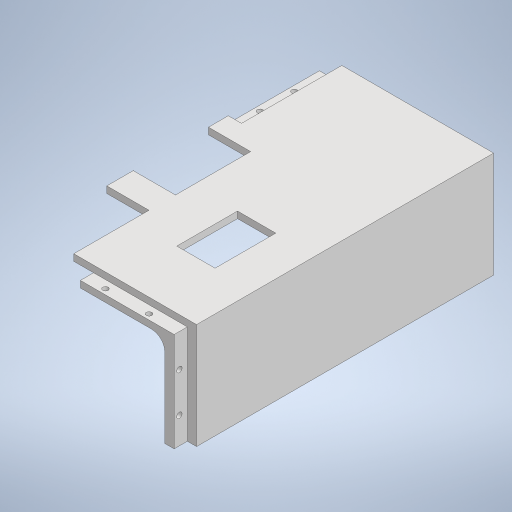
# Autodesk Inventor part: top_4
Saved by Autodesk Inventor 2023 (Build 270158000, 158)
## iProperties
Created: 2024-04-26
Part Number: top_4
Material: 常规
Document SubType Name: Modeling
Designer: Nitrene.P.L
Density: 1 g/cm^3
Appearance: 默认
Author: Nitrene.P.L
Autodesk Inventor part; units mm, degrees
ref_plane "YZ Plane" through (0, 0, 0) normal (1, 0, 0) x (0, 1, 0)
ref_plane "XZ Plane" through (0, 0, 0) normal (0, 1, 0) x (-1, 0, 0)
ref_plane "XY Plane" through (0, 0, 0) normal (0, 0, 1) x (1, 0, 0)
sketch "草图7" plane through (0, 0, 0) normal (0, 1, 0) x (-1, 0, 0)
  line L0 (125, 235) -> (-125, 235)
  line L1 (-125, 235) -> (-125, -235)
  line L2 (-125, -235) -> (125, -235)
  line L3 (125, -235) -> (125, 235)
  line L4 (0, 3) -> (0, -5)
  line L5 (3.5058, 0) -> (-3.4421, 0)
  line L6 (25, 144) -> (-32, 144)
  line L7 (-32, 144) -> (-32, 87)
  line L8 (-32, 87) -> (25, 87)
  line L9 (25, 87) -> (25, 144)
  line L10 (25, 67) -> (-32, 67)
  line L11 (-32, 67) -> (-32, 10)
  line L12 (-32, 10) -> (25, 10)
  line L13 (25, 10) -> (25, 67)
  line L14 (25, -10) -> (-32, -10)
  line L15 (-32, -10) -> (-32, -67)
  line L16 (-32, -67) -> (25, -67)
  line L17 (25, -67) -> (25, -10)
  line L18 (25, -87) -> (-32, -87)
  line L19 (-32, -87) -> (-32, -144)
  line L20 (-32, -144) -> (25, -144)
  line L21 (25, -144) -> (25, -87)
  line L22 (-66, 100) -> (-95, 100)
  line L23 (-95, 100) -> (-95, 54)
  line L24 (-95, 54) -> (-66, 54)
  line L25 (-66, 54) -> (-66, 100)
  line L26 (-66, -54) -> (-95, -54)
  line L27 (-95, -54) -> (-95, -100)
  line L28 (-95, -100) -> (-66, -100)
  line L29 (-66, -100) -> (-66, -54)
  line L30 (100, 15) -> (70, 15)
  line L31 (70, 15) -> (70, -15)
  line L32 (70, -15) -> (100, -15)
  line L33 (100, -15) -> (100, 15)
  circle A0 centre (65, 182) radius 10
  circle A1 centre (65, -182) radius 10
  circle A2 centre (65, 182) radius 15
  circle A3 centre (80, 182) radius 1.5
  circle A4 centre (57.5, 194.9904) radius 1.5
  circle A5 centre (57.5, 169.0096) radius 1.5
  line L34 (125, 235) -> (0, 235)
  line L35 (0, 235) -> (0, 0)
  line L36 (0, 0) -> (125, 0)
  line L37 (125, 0) -> (125, 235)
  line L38 (-125, 235) -> (0, 235)
  line L39 (0, 235) -> (0, 0)
  line L40 (0, 0) -> (-125, 0)
  line L41 (-125, 0) -> (-125, 235)
  line L42 (-125, -235) -> (0, -235)
  line L43 (0, -235) -> (0, 0)
  line L44 (0, 0) -> (-125, 0)
  line L45 (-125, 0) -> (-125, -235)
  line L46 (125, -235) -> (0, -235)
  line L47 (0, -235) -> (0, 0)
  line L48 (0, 0) -> (125, 0)
  line L49 (125, 0) -> (125, -235)
  circle A6 centre (65, -182) radius 15
  circle A7 centre (80, -182) radius 1.5
  circle A8 centre (57.5, -169.0096) radius 1.5
  circle A9 centre (57.5, -194.9904) radius 1.5
  point P0 (0, -87)
  point P1 (0, -67)
  point P2 (0, -10)
  point P3 (0, -235)
  point P4 (0, -144)
  dimension "d115" = 30
  dimension "d118" = 30
  dimension "d84" = 470
  dimension "d85" = 250
  dimension "d86" = 57
  dimension "d87" = 57
  dimension "d88" = 57
  dimension "d89" = 57
  dimension "d90" = 57
  dimension "d91" = 57
  dimension "d92" = 57
  dimension "d93" = 57
  dimension "d94" = 91
  dimension "d95" = 20
  dimension "d96" = 20
  dimension "d97" = 20
  dimension "d98" = 93
  dimension "d99" = 29
  dimension "d100" = 46
  dimension "d101" = 46
  dimension "d102" = 135
  dimension "d103" = 108
  dimension "d104" = 30
  dimension "d105" = 30
  dimension "d106" = 30
  dimension "d107" = 25
  dimension "d108" = 220
  dimension "d109" = 20
  dimension "d110" = 53
  dimension "d111" = 60
  dimension "d112" = 20
  dimension "d113" = 53
  dimension "d114" = 60
  dimension "d116" = 3
  dimension "d117" = 360
  dimension "d119" = 3
  dimension "d120" = 360
  constraints: 100 end point, 24 parallel, 14 horizontal, 12 perpendicular, 8 centre point, 3 collinear, 2 coincident, 2 horizontal alignment, 2 point on line, 2 vertical, 20 other
  measures "d84" distance of L3.start L37.end
  measures "d85" distance of L37.end L1.start
  measures "d86" distance of L8.end L8.start
  measures "d87" distance of L8.start L6.end
  measures "d88" distance of L12.end L12.start
  measures "d89" distance of L12.start L10.end
  measures "d90" distance of L16.end L16.start
  measures "d91" distance of L16.start L14.end
  measures "d92" distance of L20.end L20.start
  measures "d93" distance of L20.start L19.start
  measures "d94" distance between parallel lines of L0 L6
  measures "d95" distance between parallel lines of L10 L8
  measures "d96" distance between parallel lines of L12 L14
  measures "d97" distance between parallel lines of L18 L16
  measures "d98" distance between parallel lines of L1 L7
  measures "d99" distance of L25.start L23.end
  measures "d100" distance of L23.end L22.end
  measures "d101" distance of L28.start L27.start
  measures "d102" distance between parallel lines of L0 L22
  measures "d103" distance between parallel lines of L26 L24
  measures "d104" distance between parallel lines of L1 L23
  measures "d105" distance of L33.start L31.end
  measures "d106" distance of L31.end L30.end
  measures "d107" distance between parallel lines of L3 L33
  measures "d108" distance between parallel lines of L0 L30
  measures "d109" diameter of A0
  measures "d110" distance from line of L0 A0.centre
  measures "d111" distance from line of L3 A0.centre
  measures "d112" diameter of A1
  measures "d113" distance from line of L2 A1.centre
  measures "d114" distance from line of L3 A1.centre
  measures "d116" diameter of A3
  measures "d119" diameter of A7
extrude "拉伸7" add sketch "草图7" along normal blind 10 contours L40 L5 L4 L43 L14 L15 L16 L18 L19 L20 L2 L1
sketch "草图8" plane through (0, 0, 0) normal (0, -1, 0) x (1, 0, 0)
  line L0 (0, 0) -> (125, 0) projected
  line L1 (0, -235) -> (0, -144) projected
  line L2 (47, 0) -> (0, 0)
  line L3 (0, 0) -> (0, -159)
  line L4 (0, -159) -> (47, -159)
  line L5 (47, -159) -> (47, 0)
  line L6 (32, -67) -> (32, -10) projected
  line L7 (0, -144) -> (32, -144) projected
  line L8 (111, -39) -> (47, -39)
  line L9 (47, -39) -> (47, -115)
  line L10 (47, -115) -> (111, -115)
  line L11 (111, -115) -> (111, -39)
  line L12 (95, -54) -> (66, -54) projected
  line L13 (66, -100) -> (95, -100) projected
  line L14 (95, -100) -> (95, -54) projected
  line L15 (66, -54) -> (66, -100) projected
  dimension "d123" = 15
  dimension "d124" = 15
  dimension "d125" = 15
  dimension "d126" = 15
  dimension "d127" = 16
  dimension "d128" = 19
  constraints: 16 end point, 4 parallel, 2 horizontal, 2 perpendicular, 2 point on line
  measures "d123" distance between parallel lines of L6 L5
  measures "d124" distance between parallel lines of L7 L4
  measures "d125" distance between parallel lines of L8 L12
  measures "d126" distance between parallel lines of L13 L10
  measures "d127" distance between parallel lines of L14 L11
  measures "d128" distance between parallel lines of L9 L15
extrude "拉伸8" cut sketch "草图8" against normal blind 5
sketch "草图9" plane through (0, 0, 0) normal (0, -1, 0) x (1, 0, 0)
  line L0 (125, -235) -> (0, -235) projected
  line L1 (125, 0) -> (111, 0)
  line L2 (111, 0) -> (111, -235)
  line L3 (111, -235) -> (125, -235)
  line L4 (125, -235) -> (125, 0)
  line L5 (0, -235) -> (0, -159) projected
  line L6 (125, 0) -> (125, -235) projected
  line L7 (0, -235) -> (125, -235)
  line L8 (125, -235) -> (125, -221)
  line L9 (125, -221) -> (0, -221)
  line L10 (0, -221) -> (0, -235)
  point P0 (0, 0)
  point P1 (111, -221)
  dimension "d131" = 14
  dimension "d132" = 14
  constraints: 16 end point, 4 parallel, 2 horizontal, 2 perpendicular, 2 point on line
  measures "d131" distance of L3.end L2.end
  measures "d132" distance of L8.end L7.end
extrude "拉伸9" add sketch "草图9" along normal blind 70
sketch "草图10" plane through (0, 10, 0) normal (0, 1, 0) x (1, 0, 0)
  line L0 (0, 221) -> (0, 159) projected
  line L1 (125, 235) -> (0, 235) projected
  line L2 (0, 159) -> (10, 159)
  line L3 (10, 159) -> (10, 235)
  line L4 (10, 235) -> (0, 235)
  line L5 (0, 235) -> (0, 159)
  point P0 (0, 0)
  dimension "d135" = 10
  constraints: 8 end point, 2 parallel, 1 horizontal, 1 perpendicular, 1 point on line
  measures "d135" distance of L4.end L3.end
extrude "拉伸10" cut sketch "草图10" against normal blind 5
sketch "草图11" plane through (0, 5, 0) normal (0, 1, 0) x (1, 0, 0)
  circle A0 centre (4, 179) radius 2.1
  circle A1 centre (4, 205) radius 2.1
  line L0 (0, 159) -> (0, 235) projected
  line L1 (10, 159) -> (0, 159) projected
  line L2 (125, 235) -> (10, 235) projected
  point P0 (0, 0)
  dimension "d138" = 4.2
  dimension "d139" = 4.2
  dimension "d140" = 4
  dimension "d141" = 4
  dimension "d142" = 20
  dimension "d143" = 30
  constraints: 2 centre point
  measures "d138" diameter of A0
  measures "d139" diameter of A1
  measures "d140" distance from line of L0 A0.centre
  measures "d141" distance from line of L0 A1.centre
  measures "d142" distance from line of L1 A0.centre
  measures "d143" distance from line of L2 A1.centre
extrude "拉伸11" cut sketch "草图11" against normal blind 5
sketch "草图12" plane through (125, -70, -235) normal (0, 0, -1) x (-1, 0, 0)
  line L0 (125, 0) -> (125, 75) projected
  line L1 (14, 0) -> (125, 0) projected
  line L2 (125, 75) -> (115, 75)
  line L3 (115, 75) -> (115, 0)
  line L4 (115, 0) -> (125, 0)
  line L5 (125, 0) -> (125, 75)
  point P0 (125, 70)
  dimension "d146" = 10
  constraints: 8 end point, 2 parallel, 1 horizontal, 1 perpendicular, 1 point on line
  measures "d146" distance of L4.end L3.end
extrude "拉伸12" cut sketch "草图12" against normal blind 7
sketch "草图13" plane through (125, -70, -228) normal (0, 0, -1) x (-1, 0, 0)
  circle A0 centre (121, 50) radius 2.1
  circle A1 centre (121, 20) radius 2.1
  line L0 (125, 75) -> (125, 0) projected
  line L1 (115, 0) -> (0, 0) projected
  line L2 (0, 80) -> (115, 80) projected
  point P0 (125, 70)
  dimension "d149" = 4.2
  dimension "d150" = 4.2
  dimension "d151" = 4
  dimension "d152" = 4
  dimension "d153" = 20
  dimension "d154" = 30
  constraints: 2 centre point
  measures "d149" diameter of A0
  measures "d150" diameter of A1
  measures "d151" distance from line of L0 A1.centre
  measures "d152" distance from line of L0 A0.centre
  measures "d153" distance from line of L1 A1.centre
  measures "d154" distance from line of A0.centre L2
extrude "拉伸13" cut sketch "草图13" against normal blind 7
fillet "圆角2" radius 10 4 edges at (111, 0, -19.5) (111, 0, -168) (55.5, 0, -221) (111, -35, -221)
sketch "草图14" plane through (0, 0, 0) normal (0, -1, 0) x (1, 0, 0)
  circle A0 centre (65, -175) radius 10
  line L0 (125, -235) -> (125, 0) projected
  line L1 (10, -235) -> (125, -235) projected
  point P0 (0, 0)
  point P1 (125, -230)
  point P2 (120, -235)
  dimension "d159" = 20
  dimension "d160" = 60
  dimension "d161" = 60
  constraints: 1 centre point
  measures "d159" diameter of A0
  measures "d160" distance from line of L0 A0.centre
  measures "d161" distance from line of L1 A0.centre
extrude "拉伸14" add sketch "草图14" along normal blind 70
fillet "圆角3" radius 10 1 edges at (55, 0, -175)
sketch "草图16" plane through (0, 10, 0) normal (0, 1, 0) x (1, 0, 0)
  line L0 (125, 0) -> (125, 235) projected
  line L1 (0, 0) -> (125, 0)
  line L2 (125, 0) -> (125, 10)
  line L3 (125, 10) -> (0, 10)
  line L4 (0, 10) -> (0, 0)
  dimension "d167" = 10
  constraints: 8 end point, 2 parallel, 1 horizontal, 1 perpendicular, 1 point on line
  measures "d167" distance between parallel lines of L1 L3
extrude "拉伸16" cut sketch "草图16" against normal blind 5
sketch "草图17" plane through (0, 5, 0) normal (0, 1, 0) x (1, 0, 0)
  circle A0 centre (62, 4) radius 2.1
  circle A1 centre (95, 4) radius 2.1
  line L0 (125, 0) -> (47, 0) projected
  line L1 (32, 67) -> (32, 10) projected
  line L2 (125, 10) -> (125, 235) projected
  point P0 (0, 0)
  dimension "d170" = 4.2
  dimension "d171" = 4.2
  dimension "d172" = 4
  dimension "d173" = 4
  dimension "d174" = 30
  dimension "d175" = 30
  constraints: 2 centre point
  measures "d170" diameter of A0
  measures "d171" diameter of A1
  measures "d172" distance from line of L0 A0.centre
  measures "d173" distance from line of L0 A1.centre
  measures "d174" distance from line of L1 A0.centre
  measures "d175" distance from line of L2 A1.centre
extrude "拉伸17" cut sketch "草图17" against normal blind 5
sketch "草图18" plane through (125, -70, -235) normal (1, 0, 0) x (0, 0, -1)
  line L0 (-235, 60) -> (-235, 0) projected
  line L1 (-225, 75) -> (-235, 75)
  line L2 (-235, 75) -> (-235, 0)
  line L3 (-235, 0) -> (-225, 0)
  line L4 (-225, 0) -> (-225, 75)
  point P0 (-235, 70)
  constraints: 8 end point, 2 parallel, 1 horizontal, 1 perpendicular
extrude "拉伸18" cut sketch "草图18" against normal blind 7
sketch "草图19" plane through (118, -70, -235) normal (1, 0, 0) x (0, 0, -1)
  circle A0 centre (-231, 50) radius 2.1
  circle A1 centre (-231, 20) radius 2.1
  line L0 (-235, 0) -> (-235, 75) projected
  line L1 (0, 0) -> (-225, 0) projected
  line L2 (-225, 80) -> (0, 80) projected
  point P0 (-235, 70)
  dimension "d180" = 4.2
  dimension "d181" = 4.2
  dimension "d182" = 4
  dimension "d183" = 4
  dimension "d184" = 20
  dimension "d185" = 30
  constraints: 2 centre point
  measures "d180" diameter of A0
  measures "d181" diameter of A1
  measures "d182" distance from line of L0 A0.centre
  measures "d183" distance from line of L0 A1.centre
  measures "d184" distance from line of L1 A1.centre
  measures "d185" distance from line of L2 A0.centre
extrude "拉伸19" cut sketch "草图19" against normal blind 7
